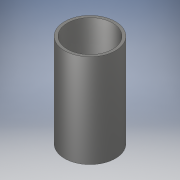
# Autodesk Inventor part: Mug
Saved by Autodesk Inventor 2019 (Build 230136000, 136)
## iProperties
Created: 2020-10-30
Part Number: Mug
Material: Aluminum 6061
Document SubType Name: Modeling
Designer: Mike
Density: 2.7 g/cm^3
Appearance: Anodized - Light Gray
Author: Mike
Autodesk Inventor part; units mm, degrees
ref_plane "YZ Plane" through (0, 0, 0) normal (1, 0, 0) x (0, 1, 0)
ref_plane "XZ Plane" through (0, 0, 0) normal (0, 1, 0) x (-1, 0, 0)
ref_plane "XY Plane" through (0, 0, 0) normal (0, 0, 1) x (1, 0, 0)
sketch "Sketch1" plane through (0, 0, 0) normal (0, 0, 1) x (1, 0, 0)
  line L0 (0, 0) -> (-25, 0)
  line L1 (-25, 0) -> (-25, 100)
  line L2 (-25, 100) -> (-28, 100)
  line L3 (-28, 100) -> (-28, -3)
  line L4 (-28, -3) -> (0, -3)
  line L5 (0, -3) -> (0, 0)
  dimension "d0" = 25
  dimension "d1" = 100
  dimension "d2" = 3
  dimension "d3" = 3
  constraints: 12 end point, 5 perpendicular, 1 horizontal
  measures "d0" distance of L0.start L0.end
  measures "d1" distance of L0.end L1.end
  measures "d2" distance of L1.end L2.end
  measures "d3" distance between parallel lines of L0 L4
revolve "Revolution1" add sketch "Sketch1" angle 360 about axis through (0, -3, 0) along (0, 1, 0)
equation "\"d3\" = d2"
body "Solid1"
